2.5mm bottom thick (Autodesk Fusion 360 design; units mm, degrees)
Autodesk Fusion 360 part; units mm, degrees
note: some values were not read from the file. Chosen so that the rebuilt part matches the saved one: which bodies a step acts on. Set by a fixed rule: which sketch regions a step uses.
sketch "Sketch1" plane through (0, 0, 0) normal (0, 0, 1) x (1, 0, 0)
  line L0 (-36.0939, 0.2498) -> (0, 0) construction
  line L1 (0, 0) -> (0.1129, 16.3059) construction
  line L2 (0.1129, 16.3059) -> (-35.9811, 16.5557) construction
  line L3 (-35.9811, 16.5557) -> (-36.0939, 0.2498) construction
  dimension "d1" = 2.5
  text T0 "2.5 mm bottom thick" font "Arial" height 2.5 align right bottom in box 36.0948 x 16.3063 at (-36.0939, 0.2498) x (0.999976, -0.006921) y (0.006921, 0.999976) spacing 1
  constraint coincident L0.end
extrude "Extrude1" add sketch "Sketch1" along normal blind 1 text T0 makes body 1 at (-25.2642, 1.0918, 0) makes body 2 at (-27.5614, 2.5589, 0) makes body 3 at (-30.7718, 0.213, 0.6667) makes body 4 at (-12.7516, 1.1189, 0) makes body 5 at (-14.3296, 1.3185, 0.3333) makes body 6 at (-13.3592, 1.3118, 0.3333) makes body 7 at (-22.355, 1.0716, 0) makes body 8 at (-29.168, 0.3184, 0.3333) makes body 9 at (-18.5801, 0.9619, 0.3333) makes body 10 at (-10.7079, 0.991, 0) makes body 11 at (-3.0968, 0.379, 0) makes body 12 at (-16.6345, 1.1458, 0) makes body 13 at (-5.961, 0.8746, 0.3333) makes body 14 at (-3.7116, 0.6294, 0.6667) makes body 15 at (-4.0071, 2.2925, 0.3333) makes body 16 at (-6.5671, 1.2648, 0.3333) makes body 17 at (-1.4949, 0.8437, 0.3333)
sketch "Sketch2" plane through (0, 0, 0) normal (0, 0, 1) x (1, 0, 0)
  line L0 (-31.5512, 3.8666) -> (0, 3.8666)
  line L1 (0, 3.8666) -> (0, -1.8666)
  line L2 (0, -1.8666) -> (-31.5512, -1.8666)
  line L3 (-31.5512, -1.8666) -> (-31.5512, 3.8666)
  circle A0 centre (0, 1) radius 2.8666
  circle A1 centre (-31.5512, 1) radius 2.8666
  constraint horizontal L0
  constraint vertical L1
  constraint horizontal L2
  constraint vertical L3
  constraint coincident L1.end A0
  constraint tangent L2 A0
  constraint coincident L0.end A0
  constraint coincident L2.end A1
  constraint tangent L2 A1
  constraint coincident L0.start A1
extrude "Extrude2" add sketch "Sketch2" against normal blind 1 bodies 1 2 3
